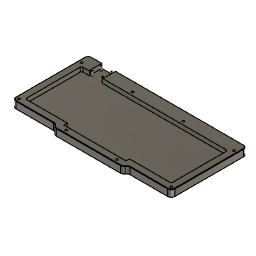
Smolboat Cutiepie Bottom Daughterboard Posts (Autodesk Fusion 360 design; units mm, degrees)
Autodesk Fusion 360 part; units mm, degrees
note: some values were not read from the file. Set by a fixed rule: which sketch regions a step uses.
sketch "Outline" plane through (0, 0, 0) normal (0, 0, 1) x (1, 0, 0)
  line L0 (25.4175, 120.057) -> (225.4425, 120.057) construction
  line L1 (225.4425, 120.057) -> (225.4425, 43.857) construction
  line L2 (225.4425, 43.857) -> (25.4175, 43.857) construction
  line L3 (25.4175, 43.857) -> (25.4175, 120.057) construction
  line L4 (125.43, 43.857) -> (125.43, 48.6195) construction
  line L5 (163.53, 58.1445) -> (87.33, 58.1445) construction
  line L6 (87.33, 58.1445) -> (87.33, 39.0945) construction
  line L7 (87.33, 39.0945) -> (163.53, 39.0945) construction
  line L8 (163.53, 39.0945) -> (163.53, 58.1445) construction
  line L9 (163.53, 58.1445) -> (87.33, 39.0945) construction
  line L10 (87.33, 58.1445) -> (163.53, 39.0945) construction
  line L11 (226.1925, 43.107) -> (24.6675, 43.107)
  line L12 (24.6675, 43.107) -> (24.6675, 120.807)
  line L13 (24.6675, 120.807) -> (226.1925, 120.807)
  line L14 (226.1925, 120.807) -> (226.1925, 43.107)
  line L15 (86.58, 58.1445) -> (86.58, 38.3445)
  line L16 (86.58, 38.3445) -> (164.28, 38.3445)
  line L17 (164.28, 38.3445) -> (164.28, 58.1445)
  line L18 (235.1925, 34.107) -> (15.6675, 34.107)
  line L19 (15.6675, 34.107) -> (15.6675, 129.807)
  line L20 (15.6675, 129.807) -> (235.1925, 129.807)
  line L21 (235.1925, 129.807) -> (235.1925, 34.107)
  line L22 (77.58, 58.1445) -> (77.58, 29.3445)
  line L23 (77.58, 29.3445) -> (173.28, 29.3445)
  line L24 (173.28, 29.3445) -> (173.28, 58.1445)
  line L25 (15.6675, 138.807) -> (15.6675, 129.807)
  line L26 (235.1925, 129.807) -> (235.1925, 138.807)
  line L27 (15.6675, 138.807) -> (235.1925, 138.807)
  line L28 (25.4175, 120.057) -> (44.4675, 120.057)
  line L29 (44.4675, 120.057) -> (44.4675, 101.007)
  line L30 (44.4675, 101.007) -> (25.4175, 101.007)
  line L31 (25.4175, 101.007) -> (25.4175, 120.057)
  line L32 (25.4175, 120.057) -> (44.4675, 101.007)
  line L33 (44.4675, 120.057) -> (43.9151, 120.057)
  line L34 (25.4175, 101.007) -> (44.4675, 120.057)
  circle A0 centre (34.9425, 110.532) radius 1.5
  point P0 (125.43, 48.6195)
  dimension "d1" = 200.025
  dimension "d2" = 76.2
  dimension "d3" = 4.7625
  dimension "d4" = 76.2
  dimension "d5" = 19.05
  dimension "d6" = -0.75
  dimension "d7" = 0.75
  dimension "d8" = -9.75
  dimension "d9" = 9.75
  dimension "d10" = 9
  dimension "d39" = 9
  dimension "d40" = 19.05
  dimension "d41" = 19.05
  dimension "d42" = 3
  constraint horizontal L0
  constraint vertical L1
  constraint horizontal L2
  constraint vertical L3
  constraint midpoint L2 L4.start
  constraint perpendicular L2 L4
  constraint horizontal L5
  constraint perpendicular L5 L6
  constraint parallel L5 L7
  constraint parallel L6 L8
  constraint coincident L9 P0
  constraint coincident L10 P0
  constraint coincident P0 L4.end
  constraint vertical L25
  constraint vertical L26
  constraint horizontal L28
  constraint vertical L29
  constraint horizontal L30
  constraint vertical L31
  constraint coincident L28 L33.end
  constraint midpoint L34 A0.centre
  measures "d1" distance of L0.start L0.end
  measures "d2" distance of L0.start L2.end
  measures "d3" distance of L4.start P0
  measures "d4" distance of L6.end L7.end
  measures "d5" distance of L5.end L6.end
  measures "d10" distance of L19.end L25.start
  measures "d39" distance of L20.end L26.end
  measures "d40" distance of L0.start L28.end
  measures "d41" distance of L0.start L30.end
  measures "d42" diameter of A0
extrude "Extrude1" add sketch "Outline" along normal blind 10 contours L11 L12 L13 L14 L18 L19 L20 L21 L22 L24 | L11 L15 L16 L17 L18 L22 L24 | L18 L22 L23 L24 | L20 L25 L26 L27
extrude "Extrude2" add sketch "Outline" along normal blind 4 contours L11 L12 L13 L14 | L11 L15 L16 L17 | L31 L32 L34 A0 | L28 L32 L33 L34 A0 | L30 L32 L34 A0 | L32 L34 A0 | L32 L34 A0 | L29 L32 L34 A0 | L32 L34 A0 | L32 L34 A0
sketch "Hole Sketch" plane through (0, 0, 0) normal (0, 0, -1) x (1, 0, 0)
  line L0 (235.1925, -138.807) -> (235.1925, -34.107)
  line L1 (235.1925, -34.107) -> (173.28, -34.107)
  line L2 (173.28, -34.107) -> (173.28, -29.3445)
  line L3 (173.28, -29.3445) -> (77.58, -29.3445)
  line L4 (77.58, -29.3445) -> (77.58, -34.107)
  line L5 (77.58, -34.107) -> (15.6675, -34.107)
  line L6 (15.6675, -34.107) -> (15.6675, -138.807)
  circle A0 centre (230.6925, -38.607) radius 1.2368
  circle A1 centre (20.1675, -125.307) radius 1.5
  circle A2 centre (20.1675, -38.607) radius 1.5
  circle A3 centre (230.6925, -125.307) radius 1.5
  line L7 (15.6675, -138.807) -> (235.1925, -138.807)
  circle A4 centre (90.3425, -125.307) radius 1.5
  circle A5 centre (160.5175, -125.307) radius 1.5
  circle A6 centre (90.3425, -33.8445) radius 1.5
  circle A7 centre (160.5175, -33.8445) radius 1.5
  dimension "d21" = 4.5
  dimension "d22" = 4.5
  dimension "d28" = 3
  dimension "d31" = 3
  dimension "d32" = 4.5
  dimension "d33" = 4.5
  dimension "d34" = 4.5
  dimension "d36" = 3
  dimension "d37" = 4.5
  dimension "d47" = 3
  dimension "d48" = 3
  dimension "d49" = 210.525
  dimension "d50" = 70.175
  dimension "d51" = 70.175
  dimension "d52" = 3
  dimension "d53" = 3
  dimension "d54" = 70.175
  dimension "d55" = 70.175
  dimension "d56" = 4.5
  dimension "d57" = 4.5
  measures "d21" distance of L0 A0.centre
  measures "d22" distance of L1 A0.centre
  measures "d28" diameter of A1
  measures "d31" diameter of A2
  measures "d32" distance of L6 A2.centre
  measures "d33" distance of L5 A2.centre
  measures "d34" distance of L6 A1.centre
  measures "d36" diameter of A3
  measures "d37" distance of L0 A3.centre
  measures "d47" diameter of A4
  measures "d48" diameter of A5
  measures "d49" distance of A1.centre A3.centre
  measures "d50" distance of A1.centre A4.centre
  measures "d51" distance of A3.centre A5.centre
  measures "d52" diameter of A7
  measures "d53" diameter of A6
  measures "d54" horizontal distance of A2.centre A6.centre
  measures "d55" horizontal distance of A0.centre A7.centre
  measures "d56" distance of L3 A6.centre
  measures "d57" distance of L3 A7.centre
hole "Hole1" at (230.6925, 38.607, 0) at (20.1675, 125.307, 0) at (20.1675, 38.607, 0) at (230.6925, 125.307, 0) at (90.3425, 125.307, 0) at (160.5175, 125.307, 0) at (90.3425, 33.8445, 0) at (160.5175, 33.8445, 0) direction (0, 0, 1) diameter 3 depth 10.5 tip angle 180 countersink diameter 6 countersink angle 90
fillet "Fillet1" radius 2 8 edges at (226.1925, 120.807, 7) (24.6675, 120.807, 7) (24.6675, 43.107, 7) (86.58, 43.107, 7) (86.58, 38.3445, 7) (164.28, 38.3445, 7) (164.28, 43.107, 7) (226.1925, 43.107, 7)
fillet "Fillet2" radius 5 8 edges at (15.6675, 34.107, 5) (15.6675, 138.807, 5) (77.58, 34.107, 5) (77.58, 29.3445, 5) (173.28, 29.3445, 5) (173.28, 34.107, 5) (235.1925, 34.107, 5) (235.1925, 138.807, 5)
chamfer "Chamfer1" distance 0.5 angle 45 14 edges at (15.6675, 86.457, 10) (17.1319, 35.5715, 10) (46.6266, 34.107, 10) (75.0255, 33.4713, 10) (78.6644, 29.9803, 10) (125.43, 29.3445, 10) (172.1955, 29.9803, 10) (175.8344, 33.4713, 10) (204.2334, 34.107, 10) (233.728, 35.5715, 10) (235.1925, 86.457, 10) (233.728, 137.3426, 10) (125.43, 138.807, 10) (17.1319, 137.3426, 10)
chamfer "Chamfer2" distance 0.5 angle 45 14 edges at (46.6266, 34.107, 0) (17.1319, 35.5715, 0) (15.6675, 86.457, 0) (17.1319, 137.3426, 0) (125.43, 138.807, 0) (233.728, 137.3426, 0) (235.1925, 86.457, 0) (233.728, 35.5715, 0) (204.2334, 34.107, 0) (175.8344, 33.4713, 0) (172.1955, 29.9803, 0) (125.43, 29.3445, 0) (78.6644, 29.9803, 0) (75.0255, 33.4713, 0)
sketch "Chin Cut Sketch" plane through (0, 0, 10) normal (0, 0, 1) x (-1, 0, 0)
  arc A0 (-166.28, -43.107) -> (-164.28, -41.107) centre (-166.28, -41.107) ccw
  line L0 (-164.28, -41.107) -> (-164.28, -40.3445)
  arc A1 (-162.28, -38.3445) -> (-164.28, -40.3445) centre (-162.28, -40.3445) ccw
  line L1 (-162.28, -38.3445) -> (-88.58, -38.3445)
  arc A2 (-86.58, -40.3445) -> (-88.58, -38.3445) centre (-88.58, -40.3445) ccw
  line L2 (-86.58, -40.3445) -> (-86.58, -41.107)
  arc A3 (-86.58, -41.107) -> (-84.58, -43.107) centre (-84.58, -41.107) ccw
  line L3 (-84.58, -43.107) -> (-26.6675, -43.107)
  arc A4 (-24.6675, -45.107) -> (-26.6675, -43.107) centre (-26.6675, -45.107) ccw
  line L4 (-24.6675, -45.107) -> (-24.6675, -118.807)
  arc A5 (-26.6675, -120.807) -> (-24.6675, -118.807) centre (-26.6675, -118.807) ccw
  line L5 (-26.6675, -120.807) -> (-224.1925, -120.807)
  arc A6 (-226.1925, -118.807) -> (-224.1925, -120.807) centre (-224.1925, -118.807) ccw
  line L6 (-226.1925, -118.807) -> (-226.1925, -45.107)
  arc A7 (-224.1925, -43.107) -> (-226.1925, -45.107) centre (-224.1925, -45.107) ccw
  line L7 (-224.1925, -43.107) -> (-166.28, -43.107)
  circle A8 centre (-230.6925, -125.307) radius 1.5
  circle A9 centre (-20.1675, -125.307) radius 1.5
  circle A10 centre (-230.6925, -38.607) radius 1.5
  circle A11 centre (-20.1675, -38.607) radius 1.5
  line L8 (-16.1675, -133.807) -> (-16.1675, -39.107)
  arc A12 (-16.1675, -39.107) -> (-20.6675, -34.607) centre (-20.6675, -39.107) ccw
  line L9 (-20.6675, -34.607) -> (-72.5856, -34.607)
  arc A13 (-77.2709, -31.9877) -> (-72.5856, -34.607) centre (-72.5856, -29.107) ccw
  arc A14 (-77.2709, -31.9877) -> (-81.1043, -29.8445) centre (-81.1043, -34.3445) ccw
  line L10 (-81.1043, -29.8445) -> (-169.7556, -29.8445)
  arc A15 (-169.7556, -29.8445) -> (-173.589, -31.9877) centre (-169.7556, -34.3445) ccw
  arc A16 (-178.2743, -34.607) -> (-173.589, -31.9877) centre (-178.2743, -29.107) ccw
  line L11 (-178.2743, -34.607) -> (-230.1925, -34.607)
  arc A17 (-230.1925, -34.607) -> (-234.6925, -39.107) centre (-230.1925, -39.107) ccw
  line L12 (-234.6925, -39.107) -> (-234.6925, -133.807)
  arc A18 (-234.6925, -133.807) -> (-230.1925, -138.307) centre (-230.1925, -133.807) ccw
  line L13 (-230.1925, -138.307) -> (-20.6675, -138.307)
  arc A19 (-20.6675, -138.307) -> (-16.1675, -133.807) centre (-20.6675, -133.807) ccw
  line L14 (-125.43, -38.3445) -> (-168.28, -38.3445)
  line L15 (-125.43, -38.3445) -> (-82.58, -38.3445)
  line L16 (-168.28, -38.3445) -> (-82.58, -38.3445)
  line L17 (-82.58, -38.3445) -> (-82.58, -43.107)
  line L18 (-82.58, -43.107) -> (-168.28, -43.107)
  line L19 (-168.28, -43.107) -> (-168.28, -38.3445)
  circle A20 centre (-160.5175, -125.307) radius 1.5
  circle A21 centre (-90.3425, -125.307) radius 1.5
  circle A22 centre (-160.5175, -33.8445) radius 1.5
  circle A23 centre (-90.3425, -33.8445) radius 1.5
  dimension "d43" = 42.85
  dimension "d44" = 42.85
  constraint midpoint L1 L14.start
  constraint parallel L1 L14
  constraint parallel L1 L15
  constraint horizontal L16
  constraint vertical L17
  constraint horizontal L18
  constraint vertical L19
  constraint coincident L3 L17.end
  measures "d43" distance of L14.start L14.end
  measures "d44" distance of L14.start L15.end
extrude "Extrude3" cut sketch "Chin Cut Sketch" against normal blind 6 contours A0 L0 A1 L7 L14 L16 L18 L19 | A2 L2 A3 L3 L15 L16 L17 L18
sketch "UBD Cut Sketch" plane through (0, 0, 10) normal (0, 0, 1) x (-1, 0, 0)
  line L0 (-16.1675, -133.807) -> (-16.1675, -39.107)
  arc A0 (-16.1675, -39.107) -> (-20.6675, -34.607) centre (-20.6675, -39.107) ccw
  line L1 (-20.6675, -34.607) -> (-72.5856, -34.607)
  arc A1 (-77.2709, -31.9877) -> (-72.5856, -34.607) centre (-72.5856, -29.107) ccw
  arc A2 (-77.2709, -31.9877) -> (-81.1043, -29.8445) centre (-81.1043, -34.3445) ccw
  line L2 (-81.1043, -29.8445) -> (-169.7556, -29.8445)
  arc A3 (-169.7556, -29.8445) -> (-173.589, -31.9877) centre (-169.7556, -34.3445) ccw
  arc A4 (-178.2743, -34.607) -> (-173.589, -31.9877) centre (-178.2743, -29.107) ccw
  line L3 (-178.2743, -34.607) -> (-230.1925, -34.607)
  arc A5 (-230.1925, -34.607) -> (-234.6925, -39.107) centre (-230.1925, -39.107) ccw
  line L4 (-234.6925, -39.107) -> (-234.6925, -133.807)
  arc A6 (-234.6925, -133.807) -> (-230.1925, -138.307) centre (-230.1925, -133.807) ccw
  line L5 (-230.1925, -138.307) -> (-20.6675, -138.307)
  arc A7 (-20.6675, -138.307) -> (-16.1675, -133.807) centre (-20.6675, -133.807) ccw
  circle A8 centre (-90.3425, -33.8445) radius 1.5
  circle A9 centre (-90.3425, -125.307) radius 1.5
  circle A10 centre (-20.1675, -38.607) radius 1.5
  circle A11 centre (-230.6925, -38.607) radius 1.5
  circle A12 centre (-20.1675, -125.307) radius 1.5
  circle A13 centre (-230.6925, -125.307) radius 1.5
  circle A14 centre (-160.5175, -125.307) radius 1.5
  circle A15 centre (-160.5175, -33.8445) radius 1.5
  line L6 (-168.28, -38.3445) -> (-82.58, -38.3445)
  line L7 (-82.58, -38.3445) -> (-82.58, -43.107)
  line L8 (-82.58, -43.107) -> (-26.6675, -43.107)
  arc A16 (-24.6675, -45.107) -> (-26.6675, -43.107) centre (-26.6675, -45.107) ccw
  line L9 (-24.6675, -45.107) -> (-24.6675, -118.807)
  arc A17 (-26.6675, -120.807) -> (-24.6675, -118.807) centre (-26.6675, -118.807) ccw
  line L10 (-26.6675, -120.807) -> (-224.1925, -120.807)
  arc A18 (-226.1925, -118.807) -> (-224.1925, -120.807) centre (-224.1925, -118.807) ccw
  line L11 (-226.1925, -118.807) -> (-226.1925, -45.107)
  arc A19 (-224.1925, -43.107) -> (-226.1925, -45.107) centre (-224.1925, -45.107) ccw
  line L12 (-224.1925, -43.107) -> (-168.28, -43.107)
  line L13 (-168.28, -43.107) -> (-168.28, -38.3445)
  line L14 (-37.4675, -120.807) -> (-51.4675, -120.807) construction
  line L15 (-53.4675, -122.807) -> (-53.4675, -135.307) construction
  line L16 (-51.4675, -137.307) -> (-37.4675, -137.307) construction
  line L17 (-35.4675, -135.307) -> (-35.4675, -122.807) construction
  arc A20 (-37.4675, -137.307) -> (-35.4675, -135.307) centre (-37.4675, -135.307) ccw construction
  arc A21 (-53.4675, -135.307) -> (-51.4675, -137.307) centre (-51.4675, -135.307) ccw construction
  arc A22 (-51.4675, -120.807) -> (-53.4675, -122.807) centre (-51.4675, -122.807) ccw construction
  arc A23 (-35.4675, -122.807) -> (-37.4675, -120.807) centre (-37.4675, -122.807) ccw construction
  line L18 (-34.9675, -135.307) -> (-34.9675, -122.807)
  arc A24 (-34.9675, -122.807) -> (-37.4675, -120.307) centre (-37.4675, -122.807) ccw
  line L19 (-37.4675, -120.307) -> (-51.4675, -120.307)
  arc A25 (-51.4675, -120.307) -> (-53.9675, -122.807) centre (-51.4675, -122.807) ccw
  line L20 (-53.9675, -122.807) -> (-53.9675, -135.307)
  arc A26 (-53.9675, -135.307) -> (-51.4675, -137.807) centre (-51.4675, -135.307) ccw
  line L21 (-51.4675, -137.807) -> (-37.4675, -137.807)
  arc A27 (-37.4675, -137.807) -> (-34.9675, -135.307) centre (-37.4675, -135.307) ccw
  circle A28 centre (-37.4675, -135.307) radius 0.9
  circle A29 centre (-51.4675, -135.307) radius 0.9
  circle A30 centre (-37.4675, -122.807) radius 0.9
  circle A31 centre (-51.4675, -122.807) radius 0.9
  line L22 (-34.9675, -135.307) -> (-34.9675, -142.6214)
  line L23 (-34.9675, -142.6214) -> (-53.9675, -142.6214)
  line L24 (-53.9675, -142.6214) -> (-53.9675, -135.307)
  line L25 (-44.4675, -137.307) -> (-44.4675, -120.307) construction
  point P0 (-35.4675, -120.807)
  point P1 (-53.4675, -120.807)
  point P2 (-35.4675, -137.307)
  dimension "d91" = 18
  dimension "d92" = 16.5
  dimension "d93" = 2
  dimension "d94" = 0.5
  dimension "d95" = 29.3
  dimension "d98" = 1.8
  dimension "d99" = 1.8
  dimension "d100" = 1.8
  dimension "d101" = 1.8
  constraint horizontal L14
  constraint vertical L15
  constraint horizontal L16
  constraint vertical L17
  constraint coincident L10 P0
  constraint coincident P2 L17
  constraint coincident P2 L16
  constraint tangent L17 A20
  constraint tangent L16 A20
  constraint tangent L16 A21
  constraint tangent L15 A21
  constraint equal A20 A21
  constraint coincident P1 L15
  constraint coincident P1 L14
  constraint tangent L15 A22
  constraint tangent L14 A22
  constraint equal A20 A22
  constraint coincident P0 L14
  constraint coincident P0 L17
  constraint tangent L14 A23
  constraint tangent L17 A23
  constraint equal A20 A23
  constraint concentric A20 A28
  constraint concentric A21 A29
  constraint concentric A23 A30
  constraint concentric A22 A31
  constraint tangent A27 L22
  constraint perpendicular L5 L22
  constraint perpendicular L20 L23
  constraint tangent A26 L24
  constraint midpoint L16 L25.start
  constraint midpoint L19 L25.end
  constraint perpendicular L19 L25
  measures "d91" distance of P0 P1
  measures "d92" distance of P0 P2
  measures "d93" radius of A20
  measures "d95" distance of L9 L20
  measures "d98" diameter of A28
  measures "d99" diameter of A29
  measures "d100" diameter of A30
  measures "d101" diameter of A31
extrude "Extrude6" cut sketch "UBD Cut Sketch" against normal blind 6 contours L5 L22 L23 L24 | L5 A26 L21 A27 L22 L24 | L10 L18 A24 A25 L20 A26 L21 A27 | A28 | A29 | A30 | A31
extrude "Extrude8" add sketch "UBD Cut Sketch" against normal up to surface (6 mm away) contours A28 | A29 | A30 | A31
sketch "Sketch7" plane through (0, 0, 9) normal (0, 0, 1) x (-1, 0, 0)
  line L0 (-223.3722, -120.0367) -> (-223.0614, -120.057)
  line L1 (-223.0614, -120.057) -> (-27.7987, -120.057)
  line L2 (-27.7987, -120.057) -> (-27.4879, -120.0367)
  line L3 (-27.4879, -120.0367) -> (-27.1824, -119.9759)
  line L4 (-27.1824, -119.9759) -> (-26.8875, -119.8758)
  line L5 (-26.8875, -119.8758) -> (-26.6081, -119.738)
  line L6 (-26.6081, -119.738) -> (-26.3491, -119.565)
  line L7 (-26.3491, -119.565) -> (-26.1149, -119.3596)
  line L8 (-26.1149, -119.3596) -> (-25.9095, -119.1254)
  line L9 (-25.9095, -119.1254) -> (-25.7365, -118.8664)
  line L10 (-25.7365, -118.8664) -> (-25.5987, -118.5871)
  line L11 (-25.5987, -118.5871) -> (-25.4986, -118.2921)
  line L12 (-25.4986, -118.2921) -> (-25.4378, -117.9866)
  line L13 (-25.4378, -117.9866) -> (-25.4175, -117.6758)
  line L14 (-25.4175, -117.6758) -> (-25.4175, -46.2382)
  line L15 (-25.4175, -46.2382) -> (-25.4378, -45.9274)
  line L16 (-25.4378, -45.9274) -> (-25.4986, -45.6219)
  line L17 (-25.4986, -45.6219) -> (-25.5987, -45.327)
  line L18 (-25.5987, -45.327) -> (-25.7365, -45.0476)
  line L19 (-25.7365, -45.0476) -> (-25.9096, -44.7886)
  line L20 (-25.9096, -44.7886) -> (-26.1149, -44.5544)
  line L21 (-26.1149, -44.5544) -> (-26.3491, -44.3491)
  line L22 (-26.3491, -44.3491) -> (-26.6081, -44.176)
  line L23 (-26.6081, -44.176) -> (-26.8875, -44.0382)
  line L24 (-26.8875, -44.0382) -> (-27.1824, -43.9381)
  line L25 (-27.1824, -43.9381) -> (-27.4879, -43.8773)
  line L26 (-27.4879, -43.8773) -> (-27.7987, -43.857)
  line L27 (-27.7987, -43.857) -> (-82.5677, -43.8568)
  line L28 (-82.5677, -43.8568) -> (-82.8785, -43.8364)
  line L29 (-82.8785, -43.8364) -> (-82.8962, -43.8329)
  arc A0 (-83.3531, -43.7182) -> (-82.8962, -43.8329) centre (-83.1451, -43.8568) ccw
  line L30 (-83.3531, -43.7182) -> (-83.479, -43.6755)
  line L31 (-83.479, -43.6755) -> (-83.7583, -43.5378)
  line L32 (-83.7583, -43.5378) -> (-84.0173, -43.3647)
  line L33 (-84.0173, -43.3647) -> (-84.2515, -43.1593)
  line L34 (-84.2515, -43.1593) -> (-84.4569, -42.9251)
  line L35 (-84.4569, -42.9251) -> (-84.6299, -42.6662)
  line L36 (-84.6299, -42.6662) -> (-84.7677, -42.3868)
  line L37 (-84.7677, -42.3868) -> (-84.8678, -42.0918)
  line L38 (-84.8678, -42.0918) -> (-84.9286, -41.7863)
  line L39 (-84.9286, -41.7863) -> (-84.9489, -41.4755)
  line L40 (-84.9489, -41.4755) -> (-84.9693, -41.1647)
  line L41 (-84.9693, -41.1647) -> (-85.0301, -40.8592)
  line L42 (-85.0301, -40.8592) -> (-85.1302, -40.5643)
  line L43 (-85.1302, -40.5643) -> (-85.268, -40.2849)
  line L44 (-85.268, -40.2849) -> (-85.441, -40.0259)
  line L45 (-85.441, -40.0259) -> (-85.6464, -39.7917)
  line L46 (-85.6464, -39.7917) -> (-85.8806, -39.5864)
  line L47 (-85.8806, -39.5864) -> (-86.1396, -39.4133)
  line L48 (-86.1396, -39.4133) -> (-86.4189, -39.2755)
  line L49 (-86.4189, -39.2755) -> (-86.7139, -39.1754)
  line L50 (-86.7139, -39.1754) -> (-87.0194, -39.1146)
  line L51 (-87.0194, -39.1146) -> (-87.3302, -39.0943)
  line L52 (-87.3302, -39.0943) -> (-94.6526, -39.0943)
  line L53 (-94.6526, -39.0943) -> (-94.7246, -39.1116)
  line L54 (-94.7246, -39.1116) -> (-94.781, -39.1597)
  line L55 (-94.781, -39.1597) -> (-94.8094, -39.2282)
  line L56 (-94.8094, -39.2282) -> (-94.8035, -39.3021)
  line L57 (-94.8035, -39.3021) -> (-94.7648, -39.3653)
  line L58 (-94.7648, -39.3653) -> (-94.5546, -39.5679)
  line L59 (-94.5546, -39.5679) -> (-94.3674, -39.7921)
  line L60 (-94.3674, -39.7921) -> (-94.2054, -40.0351)
  line L61 (-94.2054, -40.0351) -> (-94.1344, -40.1715)
  arc A1 (-93.3555, -42.7328) -> (-94.1344, -40.1715) centre (-94.442, -41.6641) ccw
  line L62 (-93.3555, -42.7328) -> (-93.3058, -42.7863)
  line L63 (-93.3058, -42.7863) -> (-93.0972, -42.9522)
  line L64 (-93.0972, -42.9522) -> (-92.8664, -43.0852)
  line L65 (-92.8664, -43.0852) -> (-92.6182, -43.1824)
  line L66 (-92.6182, -43.1824) -> (-92.3584, -43.2416)
  line L67 (-92.3584, -43.2416) -> (-92.0927, -43.2615)
  line L68 (-92.0927, -43.2615) -> (-91.9909, -43.2794)
  line L69 (-91.9909, -43.2794) -> (-91.9014, -43.3311)
  line L70 (-91.9014, -43.3311) -> (-91.8349, -43.4103)
  line L71 (-91.8349, -43.4103) -> (-91.7996, -43.5074)
  line L72 (-91.7996, -43.5074) -> (-91.7996, -43.6108)
  line L73 (-91.7996, -43.6108) -> (-91.8349, -43.708)
  line L74 (-91.8349, -43.708) -> (-91.9014, -43.7871)
  line L75 (-91.9014, -43.7871) -> (-91.9909, -43.8388)
  line L76 (-91.9909, -43.8388) -> (-92.0927, -43.8568)
  line L77 (-92.0927, -43.8568) -> (-92.3899, -43.8382)
  line L78 (-92.3899, -43.8382) -> (-92.6825, -43.7826)
  line L79 (-92.6825, -43.7826) -> (-92.9659, -43.6909)
  line L80 (-92.9659, -43.6909) -> (-93.2356, -43.5646)
  line L81 (-93.2356, -43.5646) -> (-93.4874, -43.4056)
  line L82 (-93.4874, -43.4056) -> (-93.7174, -43.2164)
  line L83 (-93.7174, -43.2164) -> (-93.8553, -43.0706)
  arc A2 (-95.6485, -42.5952) -> (-93.8553, -43.0706) centre (-94.442, -41.6641) ccw
  arc A3 (-95.6485, -40.733) -> (-95.6485, -42.5952) centre (-96.8551, -41.6641) ccw
  arc A4 (-94.8524, -40.1964) -> (-95.6485, -40.733) centre (-94.442, -41.6641) ccw
  line L84 (-94.8524, -40.1964) -> (-94.9604, -40.0333)
  line L85 (-94.9604, -40.0333) -> (-95.1658, -39.7974)
  line L86 (-95.1658, -39.7974) -> (-95.4004, -39.5904)
  line L87 (-95.4004, -39.5904) -> (-95.66, -39.416)
  line L88 (-95.66, -39.416) -> (-95.9403, -39.2771)
  line L89 (-95.9403, -39.2771) -> (-96.2363, -39.1761)
  line L90 (-96.2363, -39.1761) -> (-96.5431, -39.1148)
  line L91 (-96.5431, -39.1148) -> (-96.8552, -39.0943)
  line L92 (-96.8552, -39.0943) -> (-163.5304, -39.0943)
  line L93 (-163.5304, -39.0943) -> (-163.8409, -39.1148)
  line L94 (-163.8409, -39.1148) -> (-164.1464, -39.1756)
  line L95 (-164.1464, -39.1756) -> (-164.4413, -39.2757)
  line L96 (-164.4413, -39.2757) -> (-164.7207, -39.4135)
  line L97 (-164.7207, -39.4135) -> (-164.9797, -39.5866)
  line L98 (-164.9797, -39.5866) -> (-165.2139, -39.7919)
  line L99 (-165.2139, -39.7919) -> (-165.4193, -40.0261)
  line L100 (-165.4193, -40.0261) -> (-165.5923, -40.2851)
  line L101 (-165.5923, -40.2851) -> (-165.7301, -40.5645)
  line L102 (-165.7301, -40.5645) -> (-165.8302, -40.8594)
  line L103 (-165.8302, -40.8594) -> (-165.891, -41.1649)
  line L104 (-165.891, -41.1649) -> (-165.9113, -41.4757)
  line L105 (-165.9113, -41.4757) -> (-165.9317, -41.7865)
  line L106 (-165.9317, -41.7865) -> (-165.9925, -42.092)
  line L107 (-165.9925, -42.092) -> (-166.0926, -42.387)
  line L108 (-166.0926, -42.387) -> (-166.2304, -42.6664)
  line L109 (-166.2304, -42.6664) -> (-166.4034, -42.9253)
  line L110 (-166.4034, -42.9253) -> (-166.6088, -43.1595)
  line L111 (-166.6088, -43.1595) -> (-166.843, -43.3649)
  line L112 (-166.843, -43.3649) -> (-167.102, -43.538)
  line L113 (-167.102, -43.538) -> (-167.3813, -43.6757)
  line L114 (-167.3813, -43.6757) -> (-167.6763, -43.7758)
  line L115 (-167.6763, -43.7758) -> (-167.9818, -43.8366)
  line L116 (-167.9818, -43.8366) -> (-168.2926, -43.857)
  line L117 (-168.2926, -43.857) -> (-223.0614, -43.857)
  line L118 (-223.0614, -43.857) -> (-223.3722, -43.8774)
  line L119 (-223.3722, -43.8774) -> (-223.6777, -43.9381)
  line L120 (-223.6777, -43.9381) -> (-223.9726, -44.0382)
  line L121 (-223.9726, -44.0382) -> (-224.252, -44.176)
  line L122 (-224.252, -44.176) -> (-224.511, -44.3491)
  line L123 (-224.511, -44.3491) -> (-224.7452, -44.5544)
  line L124 (-224.7452, -44.5544) -> (-224.9506, -44.7886)
  line L125 (-224.9506, -44.7886) -> (-225.1236, -45.0476)
  line L126 (-225.1236, -45.0476) -> (-225.2614, -45.327)
  line L127 (-225.2614, -45.327) -> (-225.3615, -45.6219)
  line L128 (-225.3615, -45.6219) -> (-225.4223, -45.9274)
  line L129 (-225.4223, -45.9274) -> (-225.4426, -46.2382)
  line L130 (-225.4426, -46.2382) -> (-225.4426, -117.6758)
  line L131 (-225.4426, -117.6758) -> (-225.4223, -117.9866)
  line L132 (-225.4223, -117.9866) -> (-225.3615, -118.2921)
  line L133 (-225.3615, -118.2921) -> (-225.2614, -118.587)
  line L134 (-225.2614, -118.587) -> (-225.1236, -118.8664)
  line L135 (-225.1236, -118.8664) -> (-224.9505, -119.1254)
  line L136 (-224.9505, -119.1254) -> (-224.7452, -119.3596)
  line L137 (-224.7452, -119.3596) -> (-224.511, -119.5649)
  line L138 (-224.511, -119.5649) -> (-224.252, -119.738)
  line L139 (-224.252, -119.738) -> (-223.9726, -119.8758)
  line L140 (-223.9726, -119.8758) -> (-223.6777, -119.9759)
  line L141 (-223.6777, -119.9759) -> (-223.3722, -120.0367)
  circle A5 centre (-213.3775, -48.302) radius 0.735
  circle A6 centre (-194.3275, -48.302) radius 0.735
  circle A7 centre (-175.2775, -48.302) radius 0.735
  circle A8 centre (-219.7275, -50.842) radius 0.735
  circle A9 centre (-220.9975, -53.382) radius 0.875
  circle A10 centre (-215.9175, -53.382) radius 1.9939
  circle A11 centre (-210.8375, -53.382) radius 0.875
  circle A12 centre (-200.6775, -50.842) radius 0.735
  circle A13 centre (-201.9475, -53.382) radius 0.875
  circle A14 centre (-212.1075, -55.922) radius 1.5
  circle A15 centre (-218.4575, -58.462) radius 1.5
  circle A16 centre (-199.4075, -58.462) radius 1.5
  circle A17 centre (-196.8675, -53.382) radius 1.9939
  circle A18 centre (-191.7875, -53.382) radius 0.875
  circle A19 centre (-181.6275, -50.842) radius 0.735
  circle A20 centre (-182.8975, -53.382) radius 0.875
  circle A21 centre (-177.8175, -53.382) radius 1.9939
  circle A22 centre (-193.0575, -55.922) radius 1.5
  circle A23 centre (-174.0075, -55.922) radius 1.5
  circle A24 centre (-180.3575, -58.462) radius 1.5
  arc A25 (-155.2116, -40.733) -> (-155.2116, -42.5952) centre (-156.4181, -41.6641) ccw
  arc A26 (-155.2116, -42.5952) -> (-155.2116, -40.733) centre (-154.0051, -41.6641) ccw
  circle A27 centre (-150.6713, -46.1091) radius 0.735
  circle A28 centre (-151.9413, -48.6491) radius 0.875
  circle A29 centre (-144.3213, -43.5691) radius 0.735
  circle A30 centre (-141.9401, -43.5691) radius 0.735
  circle A31 centre (-132.5421, -41.6641) radius 1.524
  circle A32 centre (-148.2901, -46.1091) radius 0.735
  arc A33 (-148.8054, -48.2062) -> (-148.8054, -49.092) centre (-149.5601, -48.6491) ccw
  arc A34 (-145.6707, -47.0497) -> (-148.8054, -48.2062) centre (-146.8613, -48.6491) ccw
  arc A35 (-142.536, -48.2062) -> (-145.6707, -47.0497) centre (-144.4801, -48.6491) ccw
  arc A36 (-142.536, -49.092) -> (-142.536, -48.2062) centre (-141.7813, -48.6491) ccw
  arc A37 (-145.6707, -50.2485) -> (-142.536, -49.092) centre (-144.4801, -48.6491) ccw
  arc A38 (-148.8054, -49.092) -> (-145.6707, -50.2485) centre (-146.8613, -48.6491) ccw
  circle A39 centre (-139.4001, -48.6491) radius 0.875
  circle A40 centre (-129.2401, -46.1091) radius 0.735
  circle A41 centre (-130.5101, -48.6491) radius 0.875
  circle A42 centre (-125.4301, -48.6491) radius 1.9939
  circle A43 centre (-172.7375, -53.382) radius 0.875
  arc A44 (-155.2116, -55.3167) -> (-155.2116, -58.4916) centre (-156.4181, -56.9041) ccw
  arc A45 (-155.2116, -58.4916) -> (-155.2116, -55.3167) centre (-154.0051, -56.9041) ccw
  circle A46 centre (-140.6701, -51.1891) radius 1.5
  circle A47 centre (-147.0201, -53.7291) radius 1.5
  circle A48 centre (-127.9701, -53.7291) radius 1.5
  circle A49 centre (-132.5421, -56.9041) radius 1.9939
  circle A50 centre (-213.3775, -67.352) radius 0.735
  circle A51 centre (-194.3275, -67.352) radius 0.735
  circle A52 centre (-175.2775, -67.352) radius 0.735
  circle A53 centre (-219.7275, -69.892) radius 0.735
  circle A54 centre (-220.9975, -72.432) radius 0.875
  circle A55 centre (-215.9175, -72.432) radius 1.9939
  circle A56 centre (-210.8375, -72.432) radius 0.875
  circle A57 centre (-200.6775, -69.892) radius 0.735
  circle A58 centre (-201.9475, -72.432) radius 0.875
  circle A59 centre (-212.1075, -74.972) radius 1.5
  circle A60 centre (-218.4575, -77.512) radius 1.5
  circle A61 centre (-199.4075, -77.512) radius 1.5
  circle A62 centre (-196.8675, -72.432) radius 1.9939
  circle A63 centre (-191.7875, -72.432) radius 0.875
  circle A64 centre (-181.6275, -69.892) radius 0.735
  circle A65 centre (-182.8975, -72.432) radius 0.875
  circle A66 centre (-177.8175, -72.432) radius 1.9939
  circle A67 centre (-193.0575, -74.972) radius 1.5
  circle A68 centre (-174.0075, -74.972) radius 1.5
  circle A69 centre (-180.3575, -77.512) radius 1.5
  circle A70 centre (-156.2275, -67.352) radius 0.735
  circle A71 centre (-137.1775, -67.352) radius 0.735
  circle A72 centre (-162.5775, -69.892) radius 0.735
  circle A73 centre (-172.7375, -72.432) radius 0.875
  circle A74 centre (-163.8475, -72.432) radius 0.875
  circle A75 centre (-158.7675, -72.432) radius 1.9939
  circle A76 centre (-153.6875, -72.432) radius 0.875
  circle A77 centre (-161.3075, -77.512) radius 1.5
  circle A78 centre (-154.9575, -74.972) radius 1.5
  circle A79 centre (-143.5275, -69.892) radius 0.735
  circle A80 centre (-144.7975, -72.432) radius 0.875
  circle A81 centre (-139.7175, -72.432) radius 1.9939
  circle A82 centre (-134.6375, -72.432) radius 0.875
  circle A83 centre (-142.2575, -77.512) radius 1.5
  circle A84 centre (-135.9075, -74.972) radius 1.5
  circle A85 centre (-118.318, -41.6641) radius 1.524
  circle A86 centre (-122.8901, -43.5691) radius 0.735
  circle A87 centre (-110.9838, -43.5691) radius 0.735
  circle A88 centre (-103.84, -43.5691) radius 0.735
  circle A89 centre (-117.3338, -46.1091) radius 0.735
  arc A90 (-119.4769, -48.5919) -> (-119.4769, -48.7063) centre (-120.3501, -48.6491) ccw
  arc A91 (-119.4769, -48.7063) -> (-119.4769, -48.5919) centre (-118.6038, -48.6491) ccw
  arc A92 (-111.7142, -47.8118) -> (-111.7142, -49.4864) centre (-113.5238, -48.6491) ccw
  arc A93 (-111.7142, -49.4864) -> (-111.7142, -47.8118) centre (-111.46, -48.6491) ccw
  circle A94 centre (-110.19, -46.1091) radius 0.735
  arc A95 (-108.1896, -47.8118) -> (-108.1896, -49.4864) centre (-108.4438, -48.6491) ccw
  arc A96 (-108.1896, -49.4864) -> (-108.1896, -47.8118) centre (-106.38, -48.6491) ccw
  circle A97 centre (-101.3, -48.6491) radius 0.875
  circle A98 centre (-91.3951, -43.8568) radius 0.25
  circle A99 centre (-90.6451, -43.8568) radius 0.25
  circle A100 centre (-89.8951, -43.8568) radius 0.25
  circle A101 centre (-89.1451, -43.8568) radius 0.25
  circle A102 centre (-88.3951, -43.8568) radius 0.25
  circle A103 centre (-87.6451, -43.8568) radius 0.25
  circle A104 centre (-86.8951, -43.8568) radius 0.25
  circle A105 centre (-86.1451, -43.8568) radius 0.25
  circle A106 centre (-85.3951, -43.8568) radius 0.25
  circle A107 centre (-84.6451, -43.8568) radius 0.25
  circle A108 centre (-83.8951, -43.8568) radius 0.25
  circle A109 centre (-77.6463, -48.3316) radius 0.735
  circle A110 centre (-121.6201, -51.1891) radius 1.5
  circle A111 centre (-102.57, -51.1891) radius 1.5
  circle A112 centre (-108.92, -53.7291) radius 1.5
  circle A113 centre (-118.318, -56.9041) radius 1.9939
  circle A114 centre (-83.9963, -50.8716) radius 0.735
  circle A115 centre (-76.8525, -50.8716) radius 0.735
  circle A116 centre (-85.2663, -53.4116) radius 0.875
  arc A117 (-78.3767, -52.5743) -> (-78.3767, -54.2489) centre (-80.1863, -53.4116) ccw
  arc A118 (-78.3767, -54.2489) -> (-78.3767, -52.5743) centre (-78.1225, -53.4116) ccw
  arc A119 (-95.6485, -55.3167) -> (-95.6485, -58.4916) centre (-96.8551, -56.9041) ccw
  arc A120 (-95.6485, -58.4916) -> (-95.6485, -55.3167) centre (-94.442, -56.9041) ccw
  circle A121 centre (-75.5825, -58.4916) radius 1.5
  circle A122 centre (-70.5025, -48.3316) radius 0.735
  circle A123 centre (-56.215, -48.3316) radius 0.735
  circle A124 centre (-51.4525, -48.3316) radius 0.735
  circle A125 centre (-34.7837, -48.3316) radius 0.735
  circle A126 centre (-32.4025, -48.3316) radius 0.735
  arc A127 (-74.8521, -52.5743) -> (-74.8521, -54.2489) centre (-75.1063, -53.4116) ccw
  arc A128 (-74.8521, -54.2489) -> (-74.8521, -52.5743) centre (-73.0425, -53.4116) ccw
  circle A129 centre (-67.9625, -53.4116) radius 0.875
  circle A130 centre (-63.835, -53.4116) radius 0.875
  circle A131 centre (-62.565, -50.8716) radius 0.735
  arc A132 (-58.1795, -51.5026) -> (-57.9334, -51.5949) centre (-58.755, -53.4116) ccw
  arc A133 (-57.9334, -51.5949) -> (-58.1795, -51.5026) centre (-57.8025, -50.8716) ccw
  circle A134 centre (-53.9925, -53.4116) radius 1.9939
  circle A135 centre (-69.2325, -55.9516) radius 1.5
  circle A136 centre (-56.5325, -58.4916) radius 1.5
  circle A137 centre (-41.1337, -50.8716) radius 0.735
  circle A138 centre (-48.9125, -53.4116) radius 0.875
  circle A139 centre (-42.4037, -53.4116) radius 0.875
  circle A140 centre (-38.7525, -50.8716) radius 0.735
  arc A141 (-39.2678, -52.9687) -> (-39.2678, -53.8545) centre (-40.0225, -53.4116) ccw
  arc A142 (-36.1331, -51.8122) -> (-39.2678, -52.9687) centre (-37.3237, -53.4116) ccw
  arc A143 (-32.9984, -52.9687) -> (-36.1331, -51.8122) centre (-34.9425, -53.4116) ccw
  arc A144 (-32.9984, -53.8545) -> (-32.9984, -52.9687) centre (-32.2437, -53.4116) ccw
  arc A145 (-36.1331, -55.011) -> (-32.9984, -53.8545) centre (-34.9425, -53.4116) ccw
  arc A146 (-39.2678, -53.8545) -> (-36.1331, -55.011) centre (-37.3237, -53.4116) ccw
  circle A147 centre (-29.8625, -53.4116) radius 0.875
  circle A148 centre (-50.1825, -55.9516) radius 1.5
  circle A149 centre (-31.1325, -55.9516) radius 1.5
  circle A150 centre (-37.4825, -58.4916) radius 1.5
  circle A151 centre (-108.6025, -67.352) radius 0.735
  circle A152 centre (-89.5525, -67.352) radius 0.735
  circle A153 centre (-114.9525, -69.892) radius 0.735
  circle A154 centre (-116.2225, -72.432) radius 0.875
  circle A155 centre (-111.1425, -72.432) radius 1.9939
  circle A156 centre (-106.0625, -72.432) radius 0.875
  circle A157 centre (-113.6825, -77.512) radius 1.5
  circle A158 centre (-107.3325, -74.972) radius 1.5
  circle A159 centre (-95.9025, -69.892) radius 0.735
  circle A160 centre (-97.1725, -72.432) radius 0.875
  circle A161 centre (-92.0925, -72.432) radius 1.9939
  circle A162 centre (-76.8525, -69.892) radius 0.735
  circle A163 centre (-87.0125, -72.432) radius 0.875
  circle A164 centre (-78.1225, -72.432) radius 0.875
  circle A165 centre (-88.2825, -74.972) radius 1.5
  circle A166 centre (-94.6325, -77.512) radius 1.5
  circle A167 centre (-75.5825, -77.512) radius 1.5
  circle A168 centre (-70.5025, -67.352) radius 0.735
  circle A169 centre (-51.4525, -67.352) radius 1.5
  circle A170 centre (-32.4025, -67.352) radius 1.5
  circle A171 centre (-73.0425, -72.432) radius 1.9939
  circle A172 centre (-67.9625, -72.432) radius 0.875
  circle A173 centre (-57.8025, -69.892) radius 1.5
  circle A174 centre (-59.0725, -72.432) radius 0.875
  circle A175 centre (-53.9925, -72.432) radius 1.9939
  circle A176 centre (-69.2325, -74.972) radius 1.5
  circle A177 centre (-56.5325, -77.512) radius 0.735
  circle A178 centre (-48.9125, -72.432) radius 0.875
  circle A179 centre (-40.0225, -72.432) radius 0.875
  circle A180 centre (-38.7525, -69.892) radius 1.5
  circle A181 centre (-34.9425, -72.432) radius 1.9939
  circle A182 centre (-29.8625, -72.432) radius 0.875
  circle A183 centre (-50.1825, -74.972) radius 0.735
  circle A184 centre (-31.1325, -74.972) radius 0.735
  circle A185 centre (-27.2675, -75.0909) radius 0.5
  circle A186 centre (-37.4825, -77.512) radius 0.735
  circle A187 centre (-27.2675, -77.6309) radius 0.5
  circle A188 centre (-213.3775, -86.402) radius 0.735
  circle A189 centre (-194.3275, -86.402) radius 0.735
  circle A190 centre (-175.2775, -86.402) radius 0.735
  circle A191 centre (-219.7275, -88.942) radius 0.735
  circle A192 centre (-220.9975, -91.482) radius 0.875
  circle A193 centre (-215.9175, -91.482) radius 1.9939
  circle A194 centre (-210.8375, -91.482) radius 0.875
  circle A195 centre (-200.6775, -88.942) radius 0.735
  circle A196 centre (-201.9475, -91.482) radius 0.875
  circle A197 centre (-212.1075, -94.022) radius 1.5
  circle A198 centre (-218.4575, -96.562) radius 1.5
  circle A199 centre (-199.4075, -96.562) radius 1.5
  circle A200 centre (-196.8675, -91.482) radius 1.9939
  circle A201 centre (-191.7875, -91.482) radius 0.875
  circle A202 centre (-181.6275, -88.942) radius 0.735
  circle A203 centre (-182.8975, -91.482) radius 0.875
  circle A204 centre (-177.8175, -91.482) radius 1.9939
  circle A205 centre (-193.0575, -94.022) radius 1.5
  circle A206 centre (-174.0075, -94.022) radius 1.5
  circle A207 centre (-180.3575, -96.562) radius 1.5
  circle A208 centre (-156.2275, -86.402) radius 0.735
  circle A209 centre (-137.1775, -86.402) radius 0.735
  circle A210 centre (-162.5775, -88.942) radius 0.735
  circle A211 centre (-172.7375, -91.482) radius 0.875
  circle A212 centre (-163.8475, -91.482) radius 0.875
  circle A213 centre (-158.7675, -91.482) radius 1.9939
  circle A214 centre (-153.6875, -91.482) radius 0.875
  circle A215 centre (-161.3075, -96.562) radius 1.5
  circle A216 centre (-154.9575, -94.022) radius 1.5
  circle A217 centre (-143.5275, -88.942) radius 0.735
  circle A218 centre (-144.7975, -91.482) radius 0.875
  circle A219 centre (-139.7175, -91.482) radius 1.9939
  circle A220 centre (-134.6375, -91.482) radius 0.875
  circle A221 centre (-142.2575, -96.562) radius 1.5
  circle A222 centre (-135.9075, -94.022) radius 1.5
  circle A223 centre (-213.3775, -105.452) radius 0.735
  circle A224 centre (-194.3275, -105.452) radius 0.735
  circle A225 centre (-175.2775, -105.452) radius 0.735
  circle A226 centre (-219.7275, -107.992) radius 0.735
  circle A227 centre (-220.9975, -110.532) radius 0.875
  circle A228 centre (-215.9175, -110.532) radius 1.9939
  circle A229 centre (-210.8375, -110.532) radius 0.875
  circle A230 centre (-200.6775, -107.992) radius 0.735
  circle A231 centre (-201.9475, -110.532) radius 0.875
  circle A232 centre (-212.1075, -113.072) radius 1.5
  circle A233 centre (-218.4575, -115.612) radius 1.5
  circle A234 centre (-199.4075, -115.612) radius 1.5
  circle A235 centre (-196.8675, -110.532) radius 1.9939
  circle A236 centre (-191.7875, -110.532) radius 0.875
  circle A237 centre (-181.6275, -107.992) radius 0.735
  circle A238 centre (-182.8975, -110.532) radius 0.875
  circle A239 centre (-177.8175, -110.532) radius 1.9939
  circle A240 centre (-193.0575, -113.072) radius 1.5
  circle A241 centre (-174.0075, -113.072) radius 1.5
  circle A242 centre (-180.3575, -115.612) radius 1.5
  circle A243 centre (-156.2275, -105.452) radius 0.735
  circle A244 centre (-137.1775, -105.452) radius 0.735
  circle A245 centre (-162.5775, -107.992) radius 0.735
  circle A246 centre (-172.7375, -110.532) radius 0.875
  circle A247 centre (-163.8475, -110.532) radius 0.875
  circle A248 centre (-158.7675, -110.532) radius 1.9939
  circle A249 centre (-153.6875, -110.532) radius 0.875
  circle A250 centre (-161.3075, -115.612) radius 1.5
  circle A251 centre (-154.9575, -113.072) radius 1.5
  circle A252 centre (-143.5275, -107.992) radius 0.735
  circle A253 centre (-144.7975, -110.532) radius 0.875
  circle A254 centre (-139.7175, -110.532) radius 1.9939
  circle A255 centre (-134.6375, -110.532) radius 0.875
  circle A256 centre (-142.2575, -115.612) radius 1.5
  circle A257 centre (-135.9075, -113.072) radius 1.5
  circle A258 centre (-108.6025, -86.402) radius 0.735
  circle A259 centre (-89.5525, -86.402) radius 0.735
  circle A260 centre (-114.9525, -88.942) radius 0.735
  circle A261 centre (-116.2225, -91.482) radius 0.875
  circle A262 centre (-111.1425, -91.482) radius 1.9939
  circle A263 centre (-106.0625, -91.482) radius 0.875
  circle A264 centre (-113.6825, -96.562) radius 1.5
  circle A265 centre (-107.3325, -94.022) radius 1.5
  circle A266 centre (-95.9025, -88.942) radius 0.735
  circle A267 centre (-97.1725, -91.482) radius 0.875
  circle A268 centre (-92.0925, -91.482) radius 1.9939
  circle A269 centre (-76.8525, -88.942) radius 0.735
  circle A270 centre (-87.0125, -91.482) radius 0.875
  circle A271 centre (-78.1225, -91.482) radius 0.875
  circle A272 centre (-88.2825, -94.022) radius 1.5
  circle A273 centre (-94.6325, -96.562) radius 1.5
  circle A274 centre (-75.5825, -96.562) radius 1.5
  circle A275 centre (-70.5025, -86.402) radius 0.735
  circle A276 centre (-51.4525, -86.402) radius 0.735
  circle A277 centre (-45.7426, -81.8725) radius 0.15
  circle A278 centre (-45.7426, -83.1475) radius 0.15
  circle A279 centre (-44.4676, -81.8725) radius 0.15
  circle A280 centre (-43.1926, -81.8725) radius 0.15
  circle A281 centre (-44.4676, -83.1475) radius 0.15
  circle A282 centre (-43.1926, -83.1475) radius 0.15
  circle A283 centre (-27.2675, -80.1709) radius 0.5
  circle A284 centre (-27.2675, -82.7109) radius 0.5
  circle A285 centre (-45.7426, -84.4225) radius 0.15
  circle A286 centre (-44.4676, -84.4225) radius 0.15
  circle A287 centre (-43.1926, -84.4225) radius 0.15
  circle A288 centre (-27.2675, -85.2509) radius 0.5
  circle A289 centre (-32.4025, -86.402) radius 0.735
  circle A290 centre (-73.0425, -91.482) radius 1.9939
  circle A291 centre (-67.9625, -91.482) radius 0.875
  circle A292 centre (-57.8025, -88.942) radius 0.735
  circle A293 centre (-59.0725, -91.482) radius 0.875
  circle A294 centre (-53.9925, -91.482) radius 1.9939
  circle A295 centre (-69.2325, -94.022) radius 1.5
  circle A296 centre (-56.5325, -96.562) radius 1.5
  circle A297 centre (-48.9125, -91.482) radius 0.875
  circle A298 centre (-40.0225, -91.482) radius 0.875
  circle A299 centre (-38.7525, -88.942) radius 0.735
  circle A300 centre (-34.9425, -91.482) radius 1.9939
  circle A301 centre (-29.8625, -91.482) radius 0.875
  circle A302 centre (-50.1825, -94.022) radius 1.5
  circle A303 centre (-31.1325, -94.022) radius 1.5
  circle A304 centre (-37.4825, -96.562) radius 1.5
  circle A305 centre (-108.6025, -105.452) radius 0.735
  circle A306 centre (-89.5525, -105.452) radius 0.735
  circle A307 centre (-83.1877, -106.5771) radius 0.3
  circle A308 centre (-81.9177, -106.5771) radius 0.3
  circle A309 centre (-114.9525, -107.992) radius 0.735
  circle A310 centre (-116.2225, -110.532) radius 0.875
  circle A311 centre (-111.1425, -110.532) radius 1.9939
  circle A312 centre (-106.0625, -110.532) radius 0.875
  circle A313 centre (-113.6825, -115.612) radius 1.5
  circle A314 centre (-107.3325, -113.072) radius 1.5
  circle A315 centre (-95.9025, -107.992) radius 0.735
  circle A316 centre (-97.1725, -110.532) radius 0.875
  circle A317 centre (-92.0925, -110.532) radius 1.9939
  circle A318 centre (-76.8525, -107.992) radius 0.735
  circle A319 centre (-87.0125, -110.532) radius 0.875
  circle A320 centre (-78.1225, -110.532) radius 0.875
  circle A321 centre (-88.2825, -113.072) radius 1.5
  circle A322 centre (-94.6325, -115.612) radius 1.5
  circle A323 centre (-75.5825, -115.612) radius 1.5
  circle A324 centre (-70.5025, -105.452) radius 0.735
  circle A325 centre (-51.4525, -105.452) radius 0.735
  circle A326 centre (-32.4025, -105.452) radius 0.735
  circle A327 centre (-73.0425, -110.532) radius 1.9939
  circle A328 centre (-67.9625, -110.532) radius 0.875
  circle A329 centre (-57.8025, -107.992) radius 0.735
  circle A330 centre (-59.0725, -110.532) radius 0.875
  circle A331 centre (-53.9925, -110.532) radius 1.9939
  circle A332 centre (-69.2325, -113.072) radius 1.5
  circle A333 centre (-56.5325, -115.612) radius 1.5
  circle A334 centre (-48.9125, -110.532) radius 0.875
  circle A335 centre (-40.0225, -110.532) radius 0.875
  circle A336 centre (-38.7525, -107.992) radius 0.735
  circle A337 centre (-34.9425, -110.532) radius 1.9939
  circle A338 centre (-29.8625, -110.532) radius 0.875
  circle A339 centre (-50.1825, -113.072) radius 1.5
  circle A340 centre (-31.1325, -113.072) radius 1.5
  circle A341 centre (-37.4825, -115.612) radius 1.5
  line L142 (-34.9425, -110.532) -> (-53.9925, -110.532) construction
  line L143 (-44.4675, -110.532) -> (-44.4675, -124.0847) construction
  line L144 (-44.4675, -120.807) -> (-43.9675, -120.807)
  constraint coincident A337.centre L142.start
  constraint coincident A331.centre L142.end
  constraint midpoint L142 L143.start
  constraint perpendicular L1 L143
  constraint coincident L143 L144.start
  constraint perpendicular L143 L144
sketch "Sketch8" plane through (0, 138.807, 0) normal (0, 1, 0) x (-1, 0, 0)
  line L0 (-53.9675, 4) -> (-53.9675, 9.5)
  line L1 (-53.9675, 9.5) -> (-230.1925, 9.5)
  line L2 (-230.1925, 9.5) -> (-230.1925, 0.5)
  line L3 (-230.1925, 0.5) -> (-20.6675, 0.5)
  line L4 (-20.6675, 0.5) -> (-20.6675, 9.5)
  line L5 (-20.6675, 9.5) -> (-34.9675, 9.5)
  line L6 (-34.9675, 9.5) -> (-34.9675, 4)
  line L7 (-34.9675, 4) -> (-53.9675, 4)
  line L8 (-53.9675, 6.0421) -> (-53.9675, 5)
  line L9 (-52.9675, 4) -> (-35.9675, 4)
  line L10 (-34.9675, 5) -> (-34.9675, 7.0353)
  arc A0 (-53.9675, 5) -> (-52.9675, 4) centre (-52.9675, 5) ccw
  arc A1 (-35.9675, 4) -> (-34.9675, 5) centre (-35.9675, 5) ccw
  line L11 (-53.9675, 5) -> (-53.9675, 4)
  line L12 (-52.9675, 4) -> (-53.9675, 4)
  line L13 (-34.9675, 5) -> (-34.9675, 4)
  dimension "d102" = 1
  constraint coincident L0 L8.start
  constraint perpendicular L7 L8
  constraint coincident L6 L10.end
  constraint perpendicular L9 L10
  constraint tangent L8 A0
  constraint tangent L9 A0
  constraint tangent L9 A1
  constraint tangent L10 A1
  constraint equal A0 A1
  constraint coincident L0.start L7.end
  constraint tangent A0 L12
  constraint coincident L6.end L7.start
  constraint tangent A1 L13
  measures "d102" radius of A0
extrude "Extrude7" add sketch "Sketch8" against normal blind 1 contours L0 L7 A0 L11 L12 | L6 L7 A1 L13
chamfer "Chamfer3" distance 0.5 angle 45 5 edges at (53.9675, 138.807, 7.25) (34.9675, 138.807, 7.25) (35.2604, 138.807, 4.2929) (44.4675, 138.807, 4) (53.6746, 138.807, 4.2929)
equation "d1 = 19.05 mm * 10.5"
equation "d2 = 19.05 mm * 4"
equation "d3 = 19.05 mm * 0.25"
equation "d4 = 19.05 mm * 4"
equation "d43 = 38.850 mm + 4 mm"
equation "d50 = d49 / 3"
equation "d51 = d49 / 3"
equation "d54 = d49 / 3"
equation "d55 = d49 / 3"
equation "d95 = 0.5 mm + 0.75 mm + 9 mm + 19.05 mm"
